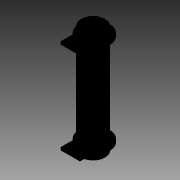
# Autodesk Inventor part: CJ2-Z_CD-Z015
Saved by Autodesk Inventor 2014 SP2 (Build 180246200, 246)
## iProperties
Created: 2020-02-04
Part Number: CJ2-Z_CD-Z015
Material: Generic
Catalog Web Link: www.cadenas.de
Description: CJ2-Z CD_PIN-Air Cylinder/Standard: Double Acting Single Rod
Vendor: SMC
Document SubType Name: Modeling
Designer: psadmin
Manufacturer: SMC
Mass: 0.470001 g
Surface Area: 4.93406 cm^2
Volume: 0.470001 cm^3
Density: 1 g/cm^3
Appearance: PSOLRGB-0-0-0
Category: PARTsolutions
Company: SMC
Title: CD-Z015
Author: Cadenas PARTsolutions
Comments: Air Cylinder/Standard: Double Acting Single Rod
PSOL_IDENT_0: {$CADENAS_DATA\23d-libs\smc_jp\actuator\standard_air_cylinder\cj2\cj2_z\parts\cj2_z_cd_pin.prj},166
PSOL_IDENT_1: {VTYP=3D},{NB=CJ2-Z_CD-Z015},{LINA=CD-Z015},{NN=CJ2-Z CD_PIN},{DATE=30.01.2020 12:57:08},{GEOMDATE=0
PSOL_IDENT_2: 9.10.2017 05:07:35},{VERSION=},{LINEID=20},{WBVAR=},{WBNUMERIC=}  {NB=CJ2-Z_CD-Z015},{LINA=CD-Z015},
PSOL_IDENT_3: {KT=DUMMY},{MODEL=CD-Z015},{BORE=16},{DD9=5 -0.030/-0.060},{DD=5.0},{D=4.8},{LL=22.7},{L=18.3},{M=1.
PSOL_IDENT_4: 5},{T=0.7},{CRIN=C-5 type for pivot}
NN: CJ2-Z CD_PIN
NT: Air Cylinder/Standard: Double Acting Single Rod
NB: CJ2-Z_CD-Z015
NBSYN: CJ2-Z_$MODEL.
LINA: CD-Z015
MODEL: CD-Z015
BORE: 16
DD9: 5 -0.030/-0.060
DD: 5
D: 4.8
LL: 22.7
L: 18.3
M: 1.5
T: 0.7
CRIN: C-5 type for pivot
SUPPLIER: SMC
ARTICLENO: CJ2-Z_CD-Z015
BOMINFO: CD-Z015
CREATOR: CADENAS GmbH
Autodesk Inventor part; units mm, degrees
sketch "Sketch_1" plane through (0, 0, 0) normal (1, 0, 0) x (0, 1, 0)
  line L0 (0, -50) -> (0, 50)
  line L1 (0, 11.35) -> (2.4, 11.35)
  line L2 (2.4, 11.35) -> (2.5, 11.25)
  line L3 (2.5, 11.25) -> (2.5, 9.85)
  line L4 (2.5, 9.85) -> (2.4, 9.85)
  line L5 (2.4, 9.85) -> (2.4, 9.15)
  line L6 (2.4, 9.15) -> (2.5, 9.15)
  line L7 (2.5, 9.15) -> (2.5, -9.15)
  line L8 (2.5, -9.15) -> (2.4, -9.15)
  line L9 (2.4, -9.15) -> (2.4, -9.85)
  line L10 (2.4, -9.85) -> (2.5, -9.85)
  line L11 (2.5, -9.85) -> (2.5, -11.25)
  line L12 (2.5, -11.25) -> (2.4, -11.35)
  line L13 (2.4, -11.35) -> (0, -11.35)
  line L14 (0, -11.35) -> (0, 11.35)
  constraints: 30 end point
revolve "Revolution1" add sketch "Sketch_1" angle 360 about axis through (0, 0, -50) along (0, 0, -1)
sketch "Sketch_4" plane through (0, 0, 9.85) normal (0, 0, 1) x (1, 0, 0)
  arc A0 (2, -2.248) -> (-2, -2.248) centre (0, 0.25) ccw
  line L0 (-2, -2.248) -> (-2, -4.75)
  line L1 (-2, -4.75) -> (2, -4.75)
  line L2 (2, -4.75) -> (2, -2.248)
  constraints: 6 end point, 2 point on circle, 1 centre point
extrude "Extrusion1" add sketch "Sketch_4" against normal blind 0.6
sketch "Sketch_5" plane through (0, 0, -9.85) normal (0, 0, 1) x (1, 0, 0)
  arc A0 (2, -2.248) -> (-2, -2.248) centre (0, 0.25) ccw
  line L0 (-2, -2.248) -> (-2, -4.75)
  line L1 (-2, -4.75) -> (2, -4.75)
  line L2 (2, -4.75) -> (2, -2.248)
  constraints: 6 end point, 2 point on circle, 1 centre point
extrude "Extrusion2" add sketch "Sketch_5" along normal blind 0.6
ref_plane "cd_XY" through (0, 0, 0) normal (1, 0, 0) x (0, 0, -1)
ref_plane "cd_YZ" through (0, 0, 0) normal (0, 0, -1) x (0, 1, 0)
ref_plane "cd_ZX" through (0, 0, 0) normal (0, 1, 0) x (1, 0, 0)
body "Solid1"
